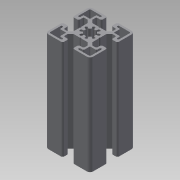
# Autodesk Inventor part: 45-4545
Saved by Autodesk Inventor 2013 (Build 170138000, 138)
## iProperties
Created: 2014-04-23
Part Number: 45-4545
Material: Generic
Document SubType Name: Modeling
Designer: Ross Bowman
Density: 1 g/cm^3
Engineer: Ross Bowman
Catalog Web Link: 8020.net
Vendor: 80/20 Inc.
Company: 80/20 Inc.
Author: Ross Bowman
Keywords: 80/20 , 8020 , T-Slot , Extrusion
Material: 6105-T5 Aluminum
Autodesk Inventor part; units mm, degrees
ref_plane "YZ Plane" through (0, 0, 0) normal (1, 0, 0) x (0, 1, 0)
ref_plane "XZ Plane" through (0, 0, 0) normal (0, 1, 0) x (-1, 0, 0)
ref_plane "XY Plane" through (0, 0, 0) normal (0, 0, 1) x (1, 0, 0)
sketch "Sketch1" plane through (0, 0, 0) normal (0, 0, 1) x (1, 0, 0)
  arc A0 (17.5, -12) -> (18.5, -11) centre (17.5, -11) ccw
  line L0 (18.5, -9) -> (18.5, -11)
  arc A1 (20.5, -9) -> (18.5, -9) centre (19.5, -9) ccw
  line L1 (20.5, -19.5) -> (20.5, -9)
  arc A2 (19.5, -20.5) -> (20.5, -19.5) centre (19.5, -19.5) ccw
  line L2 (9, -20.5) -> (19.5, -20.5)
  arc A3 (9, -18.5) -> (9, -20.5) centre (9, -19.5) ccw
  line L3 (11, -18.5) -> (9, -18.5)
  arc A4 (11, -18.5) -> (12, -17.5) centre (11, -17.5) ccw
  line L4 (12, -12.38) -> (12, -17.5)
  arc A5 (12.38, -12) -> (12, -12.38) centre (12.38, -12.38) ccw
  line L5 (17.5, -12) -> (12.38, -12)
  arc A6 (5.843, -3.7238) -> (7.2914, -3.2917) centre (6.38, -2.8802) ccw
  line L6 (4.216, -2.688) -> (5.843, -3.7238)
  arc A7 (2.6877, -4.2162) -> (4.216, -2.688) centre (0, 0) ccw
  line L7 (3.7236, -5.8429) -> (2.6877, -4.2162)
  arc A8 (3.2915, -7.2915) -> (3.7236, -5.8429) centre (2.8801, -6.3801) ccw
  arc A9 (2.8283, -7.4834) -> (3.2915, -7.2915) centre (0, 0) ccw
  arc A10 (1.4985, -6.7647) -> (2.8283, -7.4834) centre (2.4747, -6.548) ccw
  line L8 (1.0805, -4.8819) -> (1.4985, -6.7647)
  arc A11 (-1.0808, -4.8818) -> (1.0805, -4.8819) centre (0, 0) ccw
  line L9 (-1.4986, -6.7645) -> (-1.0808, -4.8818)
  arc A12 (-2.8284, -7.4833) -> (-1.4986, -6.7645) centre (-2.4749, -6.5479) ccw
  arc A13 (-3.2917, -7.2914) -> (-2.8284, -7.4833) centre (0, 0) ccw
  arc A14 (-3.7238, -5.843) -> (-3.2917, -7.2914) centre (-2.8802, -6.38) ccw
  line L10 (-2.688, -4.216) -> (-3.7238, -5.843)
  arc A15 (-4.2162, -2.6877) -> (-2.688, -4.216) centre (0, 0) ccw
  line L11 (-5.8429, -3.7236) -> (-4.2162, -2.6877)
  arc A16 (-7.2915, -3.2915) -> (-5.8429, -3.7236) centre (-6.3801, -2.8801) ccw
  arc A17 (-7.4834, -2.8283) -> (-7.2915, -3.2915) centre (0, 0) ccw
  arc A18 (-6.7647, -1.4985) -> (-7.4834, -2.8283) centre (-6.548, -2.4747) ccw
  line L12 (-4.8819, -1.0805) -> (-6.7647, -1.4985)
  arc A19 (-4.8818, 1.0808) -> (-4.8819, -1.0805) centre (0, 0) ccw
  line L13 (-6.7645, 1.4986) -> (-4.8818, 1.0808)
  arc A20 (-7.4833, 2.8284) -> (-6.7645, 1.4986) centre (-6.5479, 2.4749) ccw
  arc A21 (-7.2914, 3.2917) -> (-7.4833, 2.8284) centre (0, 0) ccw
  arc A22 (-5.843, 3.7238) -> (-7.2914, 3.2917) centre (-6.38, 2.8802) ccw
  line L14 (-4.216, 2.688) -> (-5.843, 3.7238)
  arc A23 (-2.6877, 4.2162) -> (-4.216, 2.688) centre (0, 0) ccw
  line L15 (-3.7236, 5.8429) -> (-2.6877, 4.2162)
  arc A24 (-3.2915, 7.2915) -> (-3.7236, 5.8429) centre (-2.8801, 6.3801) ccw
  arc A25 (-2.8283, 7.4834) -> (-3.2915, 7.2915) centre (0, 0) ccw
  arc A26 (-1.4985, 6.7647) -> (-2.8283, 7.4834) centre (-2.4747, 6.548) ccw
  line L16 (-1.0805, 4.8819) -> (-1.4985, 6.7647)
  arc A27 (1.0808, 4.8818) -> (-1.0805, 4.8819) centre (0, 0) ccw
  line L17 (1.4986, 6.7645) -> (1.0808, 4.8818)
  arc A28 (2.8284, 7.4833) -> (1.4986, 6.7645) centre (2.4749, 6.5479) ccw
  arc A29 (3.2917, 7.2914) -> (2.8284, 7.4833) centre (0, 0) ccw
  arc A30 (3.7238, 5.843) -> (3.2917, 7.2914) centre (2.8802, 6.38) ccw
  line L18 (2.688, 4.216) -> (3.7238, 5.843)
  arc A31 (4.2162, 2.6877) -> (2.688, 4.216) centre (0, 0) ccw
  line L19 (5.8429, 3.7236) -> (4.2162, 2.6877)
  arc A32 (7.2915, 3.2915) -> (5.8429, 3.7236) centre (6.3801, 2.8801) ccw
  arc A33 (7.4834, 2.8283) -> (7.2915, 3.2915) centre (0, 0) ccw
  arc A34 (6.7647, 1.4985) -> (7.4834, 2.8283) centre (6.548, 2.4747) ccw
  line L20 (4.8819, 1.0805) -> (6.7647, 1.4985)
  arc A35 (4.8818, -1.0808) -> (4.8819, 1.0805) centre (0, 0) ccw
  line L21 (6.7645, -1.4986) -> (4.8818, -1.0808)
  arc A36 (7.4833, -2.8284) -> (6.7645, -1.4986) centre (6.5479, -2.4749) ccw
  arc A37 (7.2914, -3.2917) -> (7.4833, -2.8284) centre (0, 0) ccw
  arc A38 (12, 12.38) -> (12.38, 12) centre (12.38, 12.38) ccw
  line L22 (12, 17.5) -> (12, 12.38)
  arc A39 (12, 17.5) -> (11, 18.5) centre (11, 17.5) ccw
  line L23 (9, 18.5) -> (11, 18.5)
  arc A40 (9, 20.5) -> (9, 18.5) centre (9, 19.5) ccw
  line L24 (19.5, 20.5) -> (9, 20.5)
  arc A41 (20.5, 19.5) -> (19.5, 20.5) centre (19.5, 19.5) ccw
  line L25 (20.5, 9) -> (20.5, 19.5)
  arc A42 (18.5, 9) -> (20.5, 9) centre (19.5, 9) ccw
  line L26 (18.5, 11) -> (18.5, 9)
  arc A43 (18.5, 11) -> (17.5, 12) centre (17.5, 11) ccw
  line L27 (12.38, 12) -> (17.5, 12)
  arc A44 (-17.5, 12) -> (-18.5, 11) centre (-17.5, 11) ccw
  line L28 (-18.5, 9) -> (-18.5, 11)
  arc A45 (-20.5, 9) -> (-18.5, 9) centre (-19.5, 9) ccw
  line L29 (-20.5, 19.5) -> (-20.5, 9)
  arc A46 (-19.5, 20.5) -> (-20.5, 19.5) centre (-19.5, 19.5) ccw
  line L30 (-9, 20.5) -> (-19.5, 20.5)
  arc A47 (-9, 18.5) -> (-9, 20.5) centre (-9, 19.5) ccw
  line L31 (-11, 18.5) -> (-9, 18.5)
  arc A48 (-11, 18.5) -> (-12, 17.5) centre (-11, 17.5) ccw
  line L32 (-12, 12.38) -> (-12, 17.5)
  arc A49 (-12.38, 12) -> (-12, 12.38) centre (-12.38, 12.38) ccw
  line L33 (-17.5, 12) -> (-12.38, 12)
  arc A50 (-12, -17.5) -> (-11, -18.5) centre (-11, -17.5) ccw
  line L34 (-9, -18.5) -> (-11, -18.5)
  arc A51 (-9, -20.5) -> (-9, -18.5) centre (-9, -19.5) ccw
  line L35 (-19.5, -20.5) -> (-9, -20.5)
  arc A52 (-20.5, -19.5) -> (-19.5, -20.5) centre (-19.5, -19.5) ccw
  line L36 (-20.5, -9) -> (-20.5, -19.5)
  arc A53 (-18.5, -9) -> (-20.5, -9) centre (-19.5, -9) ccw
  line L37 (-18.5, -11) -> (-18.5, -9)
  arc A54 (-18.5, -11) -> (-17.5, -12) centre (-17.5, -11) ccw
  line L38 (-12.38, -12) -> (-17.5, -12)
  arc A55 (-12, -12.38) -> (-12.38, -12) centre (-12.38, -12.38) ccw
  line L39 (-12, -17.5) -> (-12, -12.38)
  line L40 (-7.0516, -9.5) -> (-0.9, -9.5)
  line L41 (-0.9, -9.5) -> (0, -8.9849)
  line L42 (0, -8.9849) -> (0.9, -9.5)
  line L43 (0.9, -9.5) -> (7.0516, -9.5)
  arc A56 (7.3203, -9.6113) -> (7.0516, -9.5) centre (7.0516, -9.88) ccw
  line L44 (7.3203, -9.6113) -> (9.9387, -12.2297)
  arc A57 (10.05, -12.4984) -> (9.9387, -12.2297) centre (9.67, -12.4984) ccw
  line L45 (10.05, -12.4984) -> (10.05, -15.5)
  arc A58 (9.05, -16.5) -> (10.05, -15.5) centre (9.05, -15.5) ccw
  line L46 (9.05, -16.5) -> (6.585, -16.5)
  arc A59 (6.585, -16.5) -> (5.065, -18.02) centre (6.585, -18.02) ccw
  line L47 (5.065, -18.02) -> (5.065, -20.98)
  arc A60 (5.065, -20.98) -> (6.585, -22.5) centre (6.585, -20.98) ccw
  line L48 (6.585, -22.5) -> (19.5, -22.5)
  arc A61 (19.5, -22.5) -> (22.5, -19.5) centre (19.5, -19.5) ccw
  line L49 (22.5, -19.5) -> (22.5, -6.585)
  arc A62 (22.5, -6.585) -> (20.98, -5.065) centre (20.98, -6.585) ccw
  line L50 (20.98, -5.065) -> (18.02, -5.065)
  arc A63 (18.02, -5.065) -> (16.5, -6.585) centre (18.02, -6.585) ccw
  line L51 (16.5, -6.585) -> (16.5, -9.05)
  arc A64 (15.5, -10.05) -> (16.5, -9.05) centre (15.5, -9.05) ccw
  line L52 (15.5, -10.05) -> (12.4984, -10.05)
  arc A65 (12.2297, -9.9387) -> (12.4984, -10.05) centre (12.4984, -9.67) ccw
  line L53 (12.2297, -9.9387) -> (9.6113, -7.3203)
  arc A66 (9.5, -7.0516) -> (9.6113, -7.3203) centre (9.88, -7.0516) ccw
  line L54 (9.5, -7.0516) -> (9.5, -0.9)
  line L55 (9.5, -0.9) -> (8.9804, 0)
  line L56 (8.9804, 0) -> (9.5, 0.9)
  line L57 (9.5, 0.9) -> (9.5, 7.0516)
  arc A67 (9.6113, 7.3203) -> (9.5, 7.0516) centre (9.88, 7.0516) ccw
  line L58 (9.6113, 7.3203) -> (12.2297, 9.9387)
  arc A68 (12.4984, 10.05) -> (12.2297, 9.9387) centre (12.4984, 9.67) ccw
  line L59 (12.4984, 10.05) -> (15.5, 10.05)
  arc A69 (16.5, 9.05) -> (15.5, 10.05) centre (15.5, 9.05) ccw
  line L60 (16.5, 9.05) -> (16.5, 6.585)
  arc A70 (16.5, 6.585) -> (18.02, 5.065) centre (18.02, 6.585) ccw
  line L61 (18.02, 5.065) -> (20.98, 5.065)
  arc A71 (20.98, 5.065) -> (22.5, 6.585) centre (20.98, 6.585) ccw
  line L62 (22.5, 6.585) -> (22.5, 19.5)
  arc A72 (22.5, 19.5) -> (19.5, 22.5) centre (19.5, 19.5) ccw
  line L63 (19.5, 22.5) -> (6.585, 22.5)
  arc A73 (6.585, 22.5) -> (5.065, 20.98) centre (6.585, 20.98) ccw
  line L64 (5.065, 20.98) -> (5.065, 18.02)
  arc A74 (5.065, 18.02) -> (6.585, 16.5) centre (6.585, 18.02) ccw
  line L65 (6.585, 16.5) -> (9.05, 16.5)
  arc A75 (10.05, 15.5) -> (9.05, 16.5) centre (9.05, 15.5) ccw
  line L66 (10.05, 15.5) -> (10.05, 12.4984)
  arc A76 (9.9387, 12.2297) -> (10.05, 12.4984) centre (9.67, 12.4984) ccw
  line L67 (9.9387, 12.2297) -> (7.3203, 9.6113)
  arc A77 (7.0516, 9.5) -> (7.3203, 9.6113) centre (7.0516, 9.88) ccw
  line L68 (7.0516, 9.5) -> (0.9, 9.5)
  line L69 (0.9, 9.5) -> (0, 8.9849)
  line L70 (0, 8.9849) -> (-0.9, 9.5)
  line L71 (-0.9, 9.5) -> (-7.0516, 9.5)
  arc A78 (-7.3203, 9.6113) -> (-7.0516, 9.5) centre (-7.0516, 9.88) ccw
  line L72 (-7.3203, 9.6113) -> (-9.9387, 12.2297)
  arc A79 (-10.05, 12.4984) -> (-9.9387, 12.2297) centre (-9.67, 12.4984) ccw
  line L73 (-10.05, 12.4984) -> (-10.05, 15.5)
  arc A80 (-9.05, 16.5) -> (-10.05, 15.5) centre (-9.05, 15.5) ccw
  line L74 (-9.05, 16.5) -> (-6.585, 16.5)
  arc A81 (-6.585, 16.5) -> (-5.065, 18.02) centre (-6.585, 18.02) ccw
  line L75 (-5.065, 18.02) -> (-5.065, 20.98)
  arc A82 (-5.065, 20.98) -> (-6.585, 22.5) centre (-6.585, 20.98) ccw
  line L76 (-6.585, 22.5) -> (-19.5, 22.5)
  arc A83 (-19.5, 22.5) -> (-22.5, 19.5) centre (-19.5, 19.5) ccw
  line L77 (-22.5, 19.5) -> (-22.5, 6.585)
  arc A84 (-22.5, 6.585) -> (-20.98, 5.065) centre (-20.98, 6.585) ccw
  line L78 (-20.98, 5.065) -> (-18.02, 5.065)
  arc A85 (-18.02, 5.065) -> (-16.5, 6.585) centre (-18.02, 6.585) ccw
  line L79 (-16.5, 6.585) -> (-16.5, 9.05)
  arc A86 (-15.5, 10.05) -> (-16.5, 9.05) centre (-15.5, 9.05) ccw
  line L80 (-15.5, 10.05) -> (-12.4984, 10.05)
  arc A87 (-12.2297, 9.9387) -> (-12.4984, 10.05) centre (-12.4984, 9.67) ccw
  line L81 (-12.2297, 9.9387) -> (-9.6113, 7.3203)
  arc A88 (-9.5, 7.0516) -> (-9.6113, 7.3203) centre (-9.88, 7.0516) ccw
  line L82 (-9.5, 7.0516) -> (-9.5, 0.9)
  line L83 (-9.5, 0.9) -> (-8.9804, 0)
  line L84 (-8.9804, 0) -> (-9.5, -0.9)
  line L85 (-9.5, -0.9) -> (-9.5, -7.0516)
  arc A89 (-9.6113, -7.3203) -> (-9.5, -7.0516) centre (-9.88, -7.0516) ccw
  line L86 (-9.6113, -7.3203) -> (-12.2297, -9.9387)
  arc A90 (-12.4984, -10.05) -> (-12.2297, -9.9387) centre (-12.4984, -9.67) ccw
  line L87 (-12.4984, -10.05) -> (-15.5, -10.05)
  arc A91 (-16.5, -9.05) -> (-15.5, -10.05) centre (-15.5, -9.05) ccw
  line L88 (-16.5, -9.05) -> (-16.5, -6.585)
  arc A92 (-16.5, -6.585) -> (-18.02, -5.065) centre (-18.02, -6.585) ccw
  line L89 (-18.02, -5.065) -> (-20.98, -5.065)
  arc A93 (-20.98, -5.065) -> (-22.5, -6.585) centre (-20.98, -6.585) ccw
  line L90 (-22.5, -6.585) -> (-22.5, -19.5)
  arc A94 (-22.5, -19.5) -> (-19.5, -22.5) centre (-19.5, -19.5) ccw
  line L91 (-19.5, -22.5) -> (-6.585, -22.5)
  arc A95 (-6.585, -22.5) -> (-5.065, -20.98) centre (-6.585, -20.98) ccw
  line L92 (-5.065, -20.98) -> (-5.065, -18.02)
  arc A96 (-5.065, -18.02) -> (-6.585, -16.5) centre (-6.585, -18.02) ccw
  line L93 (-6.585, -16.5) -> (-9.05, -16.5)
  arc A97 (-10.05, -15.5) -> (-9.05, -16.5) centre (-9.05, -15.5) ccw
  line L94 (-10.05, -15.5) -> (-10.05, -12.4984)
  arc A98 (-9.9387, -12.2297) -> (-10.05, -12.4984) centre (-9.67, -12.4984) ccw
  line L95 (-9.9387, -12.2297) -> (-7.3203, -9.6113)
  arc A99 (-7.0516, -9.5) -> (-7.3203, -9.6113) centre (-7.0516, -9.88) ccw
  constraints: 200 point on circle, 192 end point, 100 centre point
extrude "Extrusion1" add sketch "Sketch1" against normal blind 100
body "Solid1"
